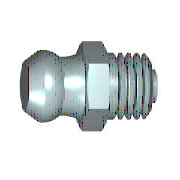
# Autodesk Inventor part: JIS B 1575 - M 6 F
Saved by Autodesk Inventor 2012 SP1 (Build 160190100, 190)
## iProperties
Created: 2011-02-07
Part Number: JIS B 1575 - M 6 F
Material: Acier doux
Description: Graisseur, conique Type A
Document SubType Name: Modeling
Standard: JIS B 1575
Designer: A.COMEAU
Standards Organization: JIS
Language: fr-FR
Size Designation: M 6 F
Categories: <MemberInstance><Categories><Category DisplayName="Autres pièces" InternalName="5aa15e00-363f-49f2-933f-16f664388e3f" Mnemonic="OTHER"><Category DisplayName="Raccords de graissage" InternalName="8c04dba7-d628-4d85-97b4-6fd8ae49030b" Mnemonic="LBCLOS"><CategoryParameter DisplayName="Filets par unité" InternalName="1d184cd2-4c2f-4bd6-9b10-c89fdadd6866" Mnemonic="thrperunit2"/><CategoryParameter DisplayName="Désignation de série de filetage" InternalName="1fe3148e-fbbd-42d5-b423-9778ea10fb80" Mnemonic="thrserdsgn2"/><CategoryParameter DisplayName="Classe de filetage" InternalName="e64f175f-656f-4cfa-b498-6f8043b7853e" Mnemonic="thrclss2"/><CategoryParameter DisplayName="Diamètre nominal" InternalName="d11a981a-7533-492a-b2a6-2f29892f1f9c" Mnemonic="nomdia2"/><CategoryParameter DisplayName="Pas de filetage" InternalName="49e7843b-de87-4b89-9c42-e94e76ef573d" Mnemonic="pitch2"/><CategoryParameter DisplayName="Désignation de filetage" InternalName="90dde9ac-ada9-413d-9d16-be72698bb726" Mnemonic="thrdesign2"/></Category></Category><Category DisplayName="Type de données" InternalName="23b78d0f-2648-40c6-8793-ca6db495c9e8" Mnemonic="DATATYPE"><CategoryParameter DisplayName="AfficherNom" InternalName="05415f3d-3907-474b-a020-eb9d644f4cf3" Mnemonic="DISPLAYNAME"/><CategoryParameter DisplayName="NomInterne" InternalName="cf1d0246-76d9-4b4a-8305-fa0409afb5c1" Mnemonic="INTERNALNAME"/><CategoryParameter DisplayName="Nom de dossier" InternalName="3f06958e-8713-4116-9be7-ed6184ecc97b" Mnemonic="FOLDERNAME"/><CategoryParameter DisplayName="Version de la famille" InternalName="914462f6-6e19-4b14-ba84-155b9680b1d0" Mnemonic="FAMILYREVISION"/><CategoryParameter DisplayName="DélimiterFormat" InternalName="bc51e27b-3422-4e78-93ef-cec197ddf230" Mnemonic="CLIPFORMAT"/><CategoryParameter DisplayName="Métrique" InternalName="e2385c5b-1ea4-4823-96a8-8de651266ec3" Mnemonic="ISMETRIC"/><CategoryParameter DisplayName="Description" InternalName="13903e3d-64b1-4950-80da-f627842ea37f" Mnemonic="DESCRIPTION"/><CategoryParameter DisplayName="OrgNorm" InternalName="8f5914e1-4693-403f-8ab5-d37768198c9d" Mnemonic="STDSORG"/><CategoryParameter DisplayName="Norme" InternalName="0c0a119c-1e12-4c84-803f-101930972f5e" Mnemonic="STANDARD"/><CategoryParameter DisplayName="Fabricant" InternalName="cd6c7a72-a28a-4e50-99a9-2c7f4e13e5ad" Mnemonic="MANUFACTURER"/><CategoryParameter DisplayName="Révision de membre" InternalName="a65d44b9-392f-4f4f-857b-e4b3d54996fe" Mnemonic="MEMBERREVISION"/><CategoryParameter DisplayName="Version standard" InternalName="91d5a463-65c2-4fde-b823-3b7fea5e8e17" Mnemonic="STANDARDREVISION"/><CategoryParameter DisplayName="Guide révision" InternalName="45a75005-10b1-4dfc-8d6d-dfe629f0b93c" Mnemonic="REVISIONGUID"/><CategoryParameter DisplayName="Désignation" InternalName="2675968c-4ce5-49e0-a4f5-552d29089031" Mnemonic="DESIGNATION"/><CategoryParameter DisplayName="NomFichier" InternalName="8b46a4cc-9585-4fed-90c3-899f57e09a73" Mnemonic="FILENAME"/><CategoryParameter DisplayName="Ligne par défaut" InternalName="2af9ec52-faaa-4026-b378-f9fa4afca842" Mnemonic="DEFAULTROW"/><Category DisplayName="Pièce" InternalName="c0e0b642-3bcb-4cc8-9e80-f96d35c4afa4" Mnemonic="PART"><CategoryParameter DisplayName="Matière" InternalName="818a152a-d3c3-49ca-80ee-df7d91421b8e" Mnemonic="MATERIAL"/><CategoryParameter DisplayName="Clé matière" InternalName="5c9a8adb-dd2b-4535-b97f-0a94a95fe41f" Mnemonic="MATERIALKEY"/><CategoryParameter DisplayName="Numéro de pièce" InternalName="016b6077-bfbe-49bd-92c9-d8d59c39c941" Mnemonic="PARTNUMBER"/><CategoryParameter DisplayName="Numéro de stock" InternalName="4dba7c1c-e26c-444e-836c-b08b433409a8" Mnemonic="STOCKNUMBER"/></Category></Category><Category DisplayName="CarteHéritée" InternalName="cd87c42b-3e48-431e-b5c0-1cbeb14dfe77" Mnemonic="LEGACYMAP"><CategoryParameter DisplayName="NomCatologue" InternalName="d99d1e27-aa94-4de2-af4c-c348882a6f4f" Mnemonic="CATALOGNAME"/><CategoryParameter DisplayName="NuméroFamille" InternalName="e705e1f4-09cb-413e-91f9-551b4188271e" Mnemonic="FAMILYNUMBER"/><CategoryParameter DisplayName="IDMembre" InternalName="8e5e0294-fc51-4c8f-b3d7-003dc5ed94f6" Mnemonic="MEMBERID"/><CategoryParameter DisplayName="ID membre CC unique" InternalName="5193edd4-b2b0-4ab4-9d54-de900eee34e0" Mnemonic="CCCOOKIE"/><CategoryParameter DisplayName="ID membre DA unique" InternalName="0918ad47-427f-4fed-ae26-24c81c58f590" Mnemonic="DACOOKIE"/><CategoryParameter DisplayName="ID de fusion11" InternalName="0ee8fb18-e2ed-4f39-96f6-1f4b5f50aa71" Mnemonic="MERGE11"/><CategoryParameter DisplayName="ID de division" InternalName="72b5c83c-be7f-45c4-ae51-9160ea6deb26" Mnemonic="SPLIT"/></Category></Categories><FamilyTemplate Id="nippla"><FamilyTemplateParameters><FamilyTemplateParameter ObjectType="kUserParameterObject" ValueType="xs:double" Id="1" ObjectReferenceKey="GUL"/><FamilyTemplateParameter ObjectType="kUserParameterObject" ValueType="xs:double" Id="2" ObjectReferenceKey="KOH"/><FamilyTemplateParameter ObjectType="kUserParameterObject" ValueType="xs:double" Id="3" ObjectReferenceKey="NLG"/><FamilyTemplateParameter ObjectType="kUserParameterObject" ValueType="xs:double" Id="4" ObjectReferenceKey="TPU"/><FamilyTemplateParameter ObjectType="kUserParameterObject" ValueType="xs:double" Id="5" ObjectReferenceKey="PHH"/><FamilyTemplateParameter ObjectType="kUserParameterObject" ValueType="xs:double" Id="6" ObjectReferenceKey="DULO"/><FamilyTemplateParameter ObjectType="kUserParameterObject" ValueType="xs:double" Id="7" ObjectReferenceKey="PTC"/><FamilyTemplateParameter ObjectType="kUserParameterObject" ValueType="xs:double" Id="8" ObjectReferenceKey="GEL"/><FamilyTemplateParameter ObjectType="kUserParameterObject" ValueType="xs:double" Id="9" ObjectReferenceKey="SW"/><FamilyTemplateParameter ObjectType="kUserParameterObject" ValueType="xs:double" Id="10" ObjectReferenceKey="THREADDIA"/><FamilyTemplateParameter ObjectType="kUserParameterObject" ValueType="xs:double" Id="11" ObjectReferenceKey="TOA"/><FamilyTemplateParameter ObjectType="kUserParameterObject" ValueType="xs:double" Id="12" ObjectReferenceKey="FAWI"/><FamilyTemplateParameter ObjectType="kUserParameterObject" ValueType="xs:double" Id="13" ObjectReferenceKey="KGB1"/><FamilyTemplateParameter ObjectType="kUserParameterObject" ValueType="xs:double" Id="14" ObjectReferenceKey="RR"/><FamilyTemplateParameter ObjectType="kUserParameterObject" ValueType="xs:double" Id="15" ObjectReferenceKey="KR"/><FamilyTemplateParameter ObjectType="kUserParameterObject" ValueType="xs:double" Id="16" ObjectReferenceKey="KGB2"/><FamilyTemplateParameter ObjectType="kUserParameterObject" ValueType="xs:double" Id="17" ObjectReferenceKey="GL"/><FamilyTemplateParameter ObjectType="kUserParameterObject" ValueType="xs:double" Id="18" ObjectReferenceKey="RBN"/><FamilyTemplateParameter ObjectType="kUserParameterObject" ValueType="xs:double" Id="19" ObjectReferenceKey="NND"/><FamilyTemplateParameter ObjectType="kUserParameterObject" ValueType="xs:double" Id="20" ObjectReferenceKey="GAL"/><FamilyTemplateParameter ObjectType="kUserParameterObject" ValueType="xs:double" Id="21" ObjectReferenceKey="VERS"/><FamilyTemplateParameter ObjectType="kUserParameterObject" ValueType="xs:double" Id="22" ObjectReferenceKey="GD1"/><FamilyTemplateParameter ObjectType="kPropertyObject" ValueType="xs:string" Id="100" ObjectReferenceKey="{32853F0F-3444-11d1-9E93-0060B03C1CA6}" SubObjectId="52"/><FamilyTemplateParameter ObjectType="kPropertyObject" ValueType="xs:string" Id="105" ObjectReferenceKey="{32853F0F-3444-11d1-9E93-0060B03C1CA6}" SubObjectId="5"/><FamilyTemplateParameter ObjectType="kPartComponentDefinitionObject" ValueType="xs:string" Id="110" SubObjectId="Material"/><FamilyTemplateParameter ObjectType="kThreadFeatureObject" ValueType="xs:structure" Id="300" ObjectReferenceKey="100200001000000063070000000000008000000000000000" SubObjectId="ThreadInfo"><FamilyTemplateParameter ObjectType="" ValueType="xs:string" Id="301" SubObjectId="ThreadDesignation"/><FamilyTemplateParameter ObjectType="" ValueType="xs:string" Id="302" SubObjectId="ThreadType"/><FamilyTemplateParameter ObjectType="" ValueType="xs:string" Id="303" SubObjectId="ThreadClass"/></FamilyTemplateParameter></FamilyTemplateParameters></FamilyTemplate><CategoryParameterMap><ParamToTemplateMap><ParamToTemplate CategoryParameter="//CategoryParameter[@InternalName='05415f3d-3907-474b-a020-eb9d644f4cf3']" ConstantValue="JIS B 1575 A - Metric"/><ParamToTemplate CategoryParameter="//CategoryParameter[@InternalName='cf1d0246-76d9-4b4a-8305-fa0409afb5c1']" ConstantValue="c8688e7c-00d7-4300-9cd4-897b0992504c"/><ParamToTemplate CategoryParameter="//CategoryParameter[@InternalName='3f06958e-8713-4116-9be7-ed6184ecc97b']" ConstantValue="JIS B 1575  A"/><ParamToTemplate CategoryParameter="//CategoryParameter[@InternalName='914462f6-6e19-4b14-ba84-155b9680b1d0']" ConstantValue="10"/><ParamToTemplate CategoryParameter="//CategoryParameter[@InternalName='bc51e27b-3422-4e78-93ef-cec197ddf230']" ConstantValue="CF_INVENTOR.STDPARTS"/><ParamToTemplate CategoryParameter="//CategoryParameter[@InternalName='e2385c5b-1ea4-4823-96a8-8de651266ec3']" ConstantValue="true"/><ParamToTemplate CategoryParameter="//CategoryParameter[@InternalName='13903e3d-64b1-4950-80da-f627842ea37f']" ConstantValue="Lubricating Nipple, coned Type A"/><ParamToTemplate CategoryParameter="//CategoryParameter[@InternalName='8f5914e1-4693-403f-8ab5-d37768198c9d']" ConstantValue="JIS"/><ParamToTemplate CategoryParameter="//CategoryParameter[@InternalName='0c0a119c-1e12-4c84-803f-101930972f5e']" ConstantValue="JIS B 1575"/><ParamToTemplate CategoryParameter="//CategoryParameter[@InternalName='cd6c7a72-a28a-4e50-99a9-2c7f4e13e5ad']" TemplateParameter="104"/><ParamToTemplate CategoryParameter="//CategoryParameter[@InternalName='91d5a463-65c2-4fde-b823-3b7fea5e8e17']" TemplateParameter="103"/><ParamToTemplate CategoryParameter="//CategoryParameter[@InternalName='45a75005-10b1-4dfc-8d6d-dfe629f0b93c']" ConstantValue="2b453dd7-f8f7-4345-b102-5654b3e566ad"/><ParamToTemplate CategoryParameter="//CategoryParameter[@InternalName='2af9ec52-faaa-4026-b378-f9fa4afca842']" ConstantValue="10"/><ParamToTemplate CategoryParameter="//CategoryParameter[@InternalName='d99d1e27-aa94-4de2-af4c-c348882a6f4f']" ConstantValue="JIS"/><ParamToTemplate CategoryParameter="//CategoryParameter[@InternalName='8b46a4cc-9585-4fed-90c3-899f57e09a73']" ConstantValue="JIS B 1575 - M 6 x 1 F"/><ParamToTemplate CategoryParameter="//CategoryParameter[@InternalName='a65d44b9-392f-4f4f-857b-e4b3d54996fe']" ConstantValue="30713309-1463-41cc-9156-af6b4ec652a7"/><ParamToTemplate CategoryParameter="//CategoryParameter[@InternalName='90dde9ac-ada9-413d-9d16-be72698bb726']" ConstantValue="M6"/><ParamToTemplate CategoryParameter="//CategoryParameter[@InternalName='e64f175f-656f-4cfa-b498-6f8043b7853e']" ConstantValue="6g"/><ParamToTemplate CategoryParameter="//CategoryParameter[@InternalName='e705e1f4-09cb-413e-91f9-551b4188271e']" ConstantValue="154"/><ParamToTemplate CategoryParameter="//CategoryParameter[@InternalName='8e5e0294-fc51-4c8f-b3d7-003dc5ed94f6']" ConstantValue="1"/><ParamToTemplate CategoryParameter="//CategoryParameter[@InternalName='2675968c-4ce5-49e0-a4f5-552d29089031']" TemplateParameter="100"/><ParamToTemplate CategoryParameter="//CategoryParameter[@InternalName='818a152a-d3c3-49ca-80ee-df7d91421b8e']" TemplateParameter="110"/><ParamToTemplate CategoryParameter="//CategoryParameter[@InternalName='d11a981a-7533-492a-b2a6-2f29892f1f9c']" TemplateParameter="19"/><ParamToTemplate CategoryParameter="//CategoryParameter[@InternalName='016b6077-bfbe-49bd-92c9-d8d59c39c941']" TemplateParameter="105"/><ParamToTemplate CategoryParameter="//CategoryParameter[@InternalName='49e7843b-de87-4b89-9c42-e94e76ef573d']" TemplateParameter="7"/><ParamToTemplate CategoryParameter="//CategoryParameter[@InternalName='1d184cd2-4c2f-4bd6-9b10-c89fdadd6866']" TemplateParameter="4"/></ParamToTemplateMap></CategoryParameterMap></MemberInstance>
Density: 1 g/cm^3
IsCustomPart: 0
Author: A.COMEAU
Autodesk Inventor part; units mm, degrees
ref_plane "YZ Plane" through (0, 0, 0) normal (1, 0, 0) x (0, 1, 0)
ref_plane "XZ Plane" through (0, 0, 0) normal (0, 1, 0) x (-1, 0, 0)
ref_plane "XY Plane" through (0, 0, 0) normal (0, 0, 1) x (1, 0, 0)
sketch "Esquisse1" plane through (0, 0, 0) normal (0, 0, 1) x (1, 0, 0)
  line L0 (-8.8, 0) -> (-8.8, 2.4)
  line L1 (-8.8, 2.4) -> (-7.335, 3.2016)
  line L2 (-8.8, 0) -> (4.7, 0)
  line L3 (4.7, 0) -> (4.7, 1.5)
  line L4 (4.7, 1.5) -> (4, 1.5)
  line L5 (4, 1.5) -> (4, 3)
  line L6 (4, 3) -> (0, 3)
  arc A0 (-4.7886, 2.8) -> (-7.335, 3.2016) centre (-6.535, 0) ccw
  line L7 (-11.5, 0) -> (7.4, 0) projected
  line L8 (0, -1.7331) -> (0, 10.3984) projected
  arc A1 (-4.7886, 2.8) -> (-3, 3.5) centre (-6.0528, 8.6653) ccw
  line L9 (-3, 3.5) -> (0, 3.5)
  line L10 (0, 3.5) -> (0, 3)
  dimension "d0" = 13.5
  dimension "d1" = 5.6
  dimension "d2" = 0.7
  dimension "d3" = 3
  dimension "d4" = 6
  dimension "d5" = 6.6
  dimension "d6" = 4.8
  dimension "d7" = 6
  dimension "d11" = 7
  dimension "d14" = 3
  dimension "d15" = 4
  dimension "d61" = 7.335
  dimension "d62" = 6.5351
  constraints: 18 end point, 5 perpendicular, 4 point on circle, 2 centre point, 2 parallel, 2 point on line, 1 collinear, 1 vertical
  measures "d0" distance between parallel lines of L0 L3
  measures "d1" diameter of A0.start L2
  measures "d2" distance between parallel lines of L3 L5
  measures "d3" diameter of L4 L2
  measures "d4" diameter of L6 L2
  measures "d6" diameter of L0.end L2
  measures "d7" radius of A1
  measures "d11" diameter of L9.start L2
  measures "d14" distance of L9.start L9.end
  measures "d15" distance between parallel lines of L5 L10
  measures "d61" distance from line of L8 L1.end
  measures "d62" distance from line of L8 A0.centre
revolve "Corps" add sketch "Esquisse1" angle 360 about axis through (-8.8, 0, 0) along (1, 0, 0)
fillet "Congé1" radius 0.2 1 edges at (-8.8, -2.4, 0)
thread "Filetage1" size "M6x1" class "6g" standard "ISO Metric profile" length 3.3866
sketch "Esquisse2" plane through (0, 0, 0) normal (1, 0, 0) x (0, 0, -1)
  circle A0 centre (0, 0) radius 3.5 projected
  line L0 (2.0207, 3.5) -> (4.0415, 0)
  line L1 (4.0415, 0) -> (2.0207, -3.5)
  line L2 (2.0207, -3.5) -> (-2.0207, -3.5)
  line L3 (-2.0207, -3.5) -> (-4.0415, 0)
  line L4 (-4.0415, 0) -> (-2.0207, 3.5)
  line L5 (-2.0207, 3.5) -> (2.0207, 3.5)
  constraints: 12 end point, 1 coincident, 1 horizontal, 1 tangent, 11 other
extrude "Tête" add sketch "Esquisse2" against normal blind 3 contours A0 L0 L1 | A0 L5 L0 | L1 L2 A0 | A0 L4 L5 | L2 L3 A0 | A0 L3 L4
sketch "Esquisse3" plane through (0, 0, 0) normal (0, 1, 0) x (-1, 0, 0)
  line L0 (2.6874, 4.0415) -> (3, 4.0415)
  line L1 (3, 4.0415) -> (3, 3.5)
  line L2 (3, 3.5) -> (2.6874, 4.0415)
  line L3 (0.3126, 4.0415) -> (0, 4.0415)
  line L4 (0, 4.0415) -> (0, 3.5)
  line L5 (0, 3.5) -> (0.3126, 4.0415)
  line L6 (3.6, 0) -> (-0.6, 0) projected
  line L7 (0, 4.0415) -> (0, 2.0207) projected
  line L8 (0, 4.0415) -> (3, 4.0415) projected
  line L9 (3, 3.0311) -> (3, 4.0415) projected
  dimension "d19" = 3.5
  dimension "d20" = 3.5
  dimension "d21" = 30
  dimension "d22" = 30
  constraints: 12 end point, 4 collinear, 3 perpendicular, 1 horizontal
  measures "d19" distance from line of L4.end L6
  measures "d20" distance from line of L1.end L6
  measures "d21" angle of L5 L4
  measures "d22" angle of L1 L2
revolve "Chanfrein1" cut sketch "Esquisse3" angle 360 about axis through (-10, 0, 0) along (1, 0, 0)
chamfer "Chanfrein2" distance 0.6135 angle 45 1 edges at (4, -3, 0) measured on face at (4, 2.4564, -0.359)
equation "\"d17\" = KOH"
equation "\"d8\" = RR"
equation "\"d9\" = NLG - GAL"
equation "\"d23\" = -0.5 * GD1 + 0.5 * NND"
equation "\"d59\" = -0.5 * GD1 + 0.5 * NND"
equation "\"d0\" = GL"
equation "\"d1\" = KGB2"
equation "\"d2\" = PHH"
equation "\"d3\" = 0.5 * NND"
equation "\"d4\" = NND"
equation "\"d5\" = KR"
equation "\"d6\" = KGB1"
equation "\"d7\" = RBN"
equation "\"d11\" = SW"
equation "\"d14\" = KOH"
equation "\"d15\" = NLG"
equation "\"d19\" = 0.5 * SW"
equation "\"d20\" = 0.5 * SW"
equation "\"NLG\" = 4"
equation "\"GL\" = 13.5"
equation "\"NND\" = 6"
equation "\"KGB1\" = 4.8"
equation "\"KGB2\" = 5.6"
equation "\"VERS\" = 0.8"
equation "\"KR\" = 6.6"
equation "\"RBN\" = 6"
equation "\"SW\" = 7"
equation "\"KOH\" = 3"
equation "\"GAL\" = 0.61345 * PTC"
equation "\"FAWI\" = 45deg"
equation "\"PHH\" = 0.7"
equation "\"GD1\" = THREADDIA - 1.2269 * PTC"
equation "\"RR\" = 0.2"
equation "\"GUL\" = 0.61345 * PTC"
equation "\"DULO\" = 1.5"
equation "\"PTC\" = 1"
equation "\"GEL\" = 4"
equation "\"THREADDIA\" = 6"
equation "\"TOA\" = 30deg"
body "Solid1"
